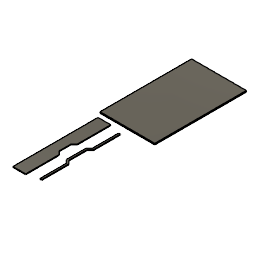
power_supply_back_cayberpunk (Autodesk Fusion 360 design; units mm, degrees)
Autodesk Fusion 360 part; units mm, degrees
sketch "Schizzo1" plane through (0, 0, 0) normal (0, 0, 1) x (1, 0, 0)
  line L0 (0, 0) -> (85, 0)
  line L1 (85, 0) -> (85, 142)
  line L2 (85, 142) -> (0, 142)
  line L3 (0, 142) -> (0, 0)
  dimension "d1" = 142
  dimension "d2" = 85
  constraint horizontal L0
  constraint vertical L1
  constraint horizontal L2
  constraint vertical L3
  constraint coincident L0.start L3.end
  measures "d1" distance of L0.start L2.end
  measures "d2" distance of L1.end L2.end
extrude "Estrusione1" add sketch "Schizzo1" along normal blind 2 makes body 1
sketch "Schizzo2" plane through (0, 0, 2) normal (0, 0, 1) x (-1, 0, 0)
  line L0 (0, -142) -> (0, 0)
  line L1 (0, 0) -> (-85, 0)
  line L2 (-85, 0) -> (-85, -142)
  line L3 (-85, -142) -> (0, -142)
  line L4 (-45, 135) -> (-42, 135)
  line L5 (-40, 60) -> (-40, 88)
  line L6 (-45, 13) -> (-45, 55)
  line L7 (-42, 135) -> (-42, 94.2426)
  line L8 (-37, 58.7574) -> (-37, 89.2426)
  line L9 (-42, 13) -> (-45, 13)
  line L10 (-20, 65) -> (-20, 83)
  line L11 (-25, 88) -> (-17.9289, 88) construction
  line L12 (-5, 140) -> (-5, 8)
  line L13 (-25, 8) -> (-25, 60)
  line L14 (-25, 140) -> (-25, 88)
  line L15 (-45, 13) -> (-42, 13)
  line L16 (-25, 140) -> (-5, 140)
  line L17 (-25, 8) -> (-25, 60)
  line L18 (-5, 8) -> (-25, 8)
  line L19 (-42, 94.2426) -> (-37, 89.2426)
  line L20 (-25, 8) -> (-25, 13)
  line L21 (-42, 53.7574) -> (-37, 58.7574)
  line L22 (-42, 13) -> (-42, 53.7574)
  line L23 (-45, 93) -> (-40, 88)
  line L24 (-25, 88) -> (-20, 83)
  line L25 (-45, 135) -> (-45, 93)
  line L26 (-45, 55) -> (-40, 60)
  line L27 (-25, 60) -> (-20, 65)
  line L28 (-25, 8) -> (-25, 60)
  line L29 (-25, 88) -> (-25, 140)
  point P0 (-5, 140)
  dimension "d16" = -3
  dimension "d17" = 132
  dimension "d18" = 52
  dimension "d19" = 52
  dimension "d20" = 7.0711
  dimension "d21" = 45
  dimension "d22" = 7.0711
  dimension "d23" = 5
  dimension "d24" = 42
  constraint horizontal L18
  constraint vertical L28
  constraint horizontal L16
  constraint vertical L12
  constraint perpendicular L14 L16
  constraint horizontal L11
  constraint perpendicular L10 L11
  constraint perpendicular L18 L20
  constraint perpendicular L9 L28
  constraint perpendicular L6 L9
  constraint perpendicular L13 L18
  constraint perpendicular L15 L22
  constraint perpendicular L4 L7
  constraint collinear L28 L29
  measures "d17" distance of L13.start L14.start
  measures "d18" distance of L14.start L11.start
  measures "d19" distance of L13.start L13.end
  measures "d20" distance of L13.end L10.start
  measures "d21" angle of L11 L24
  measures "d22" distance of L11.start L10.end
  measures "d23" distance of L13.start L20.end
  measures "d24" distance of L6.end L6.start
extrude "Estrusione2" add sketch "Schizzo2" along normal blind 1 separate body contours L4 L5 L6 L7 L8 L9 L15 L19 L21 L22 L23 L25 L26 | L10 L12 L13 L14 L16 L17 L18 L20 L24 L27 L28 L29 makes body 2 at (18.3333, -122.6667, 2) makes body 3 at (44, -40.5858, 2)
move_body "Sposta1" bodies 2 3 to x (1, 0, 0) y (0, 1, 0) z (0, 0, 1) at (0, 0, -2)
named bodies: "main", "lower", "cyber strand"
